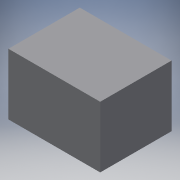
# Autodesk Inventor part: solenoid
Saved by Autodesk Inventor 2018 (Build 220112000, 112)
## iProperties
Created: 2017-05-03
Part Number: solenoid
Material: Generic
Document SubType Name: Modeling
Designer: gsegs
Density: 1 g/cm^3
Appearance: Default
Author: gsegs
Autodesk Inventor part; units mm, degrees
ref_plane "YZ Plane" through (0, 0, 0) normal (1, 0, 0) x (0, 1, 0)
ref_plane "XZ Plane" through (0, 0, 0) normal (0, 1, 0) x (-1, 0, 0)
ref_plane "XY Plane" through (0, 0, 0) normal (0, 0, 1) x (1, 0, 0)
sketch "Sketch1" plane through (0, 0, 0) normal (0, 1, 0) x (-1, 0, 0)
  line L0 (63.8432, -21.5475) -> (-50.4568, -21.5475)
  line L1 (-50.4568, -21.5475) -> (-50.4568, 67.3525)
  line L2 (-50.4568, 67.3525) -> (63.8432, 67.3525)
  line L3 (63.8432, 67.3525) -> (63.8432, -21.5475)
  point P0 (0, 0)
  dimension "d0" = 88.9
  dimension "d1" = 114.3
  constraints: 8 end point, 2 parallel, 1 horizontal, 1 perpendicular
  measures "d0" distance between parallel lines of L2 L0
  measures "d1" distance between parallel lines of L1 L3
extrude "Extrusion1" add sketch "Sketch1" along normal mid plane 76.2
body "Solid1"
